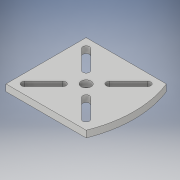
# Autodesk Inventor part: Shoddy Drilling Platform Representation
Saved by Autodesk Inventor 2018 (Build 220112000, 112)
## iProperties
Created: 2018-12-23
Part Number: Shoddy Drilling Platform Representation
Material: Generic
Document SubType Name: Modeling
Designer: Gabriel
Density: 1 g/cm^3
Appearance: Default
Author: Gabriel
Autodesk Inventor part; units mm, degrees
ref_plane "YZ Plane" through (0, 0, 0) normal (1, 0, 0) x (0, 1, 0)
ref_plane "XZ Plane" through (0, 0, 0) normal (0, 1, 0) x (-1, 0, 0)
ref_plane "XY Plane" through (0, 0, 0) normal (0, 0, 1) x (1, 0, 0)
sketch "Sketch1" plane through (0, 0, 0) normal (0, 1, 0) x (-1, 0, 0)
  line L0 (7.0481, 13.5339) -> (-297.7519, 13.5339)
  line L1 (-297.7519, 13.5339) -> (-297.7519, -291.2661)
  line L2 (-297.7519, -291.2661) -> (7.0481, -291.2661)
  line L3 (7.0481, -291.2661) -> (7.0481, 13.5339)
  arc A0 (-297.7519, 13.5339) -> (-297.7519, -291.2661) centre (83.7145, -138.8661) ccw
  point P0 (0, 0)
  dimension "d0" = 304.8
  dimension "d1" = 304.8
  constraints: 8 end point, 2 parallel, 2 point on circle, 1 centre point, 1 horizontal, 1 perpendicular
  measures "d0" distance of L2.end L1.end
  measures "d1" distance of L1.end L0.end
extrude "Extrusion1" add sketch "Sketch1" along normal blind 25.4
sketch "Sketch2" plane through (0, 25.4, 0) normal (0, 1, 0) x (1, 0, 0)
  line L0 (-7.0481, 291.2661) -> (-7.0481, -13.5339) projected
  line L1 (-7.0481, 138.8661) -> (145.3519, 138.8661)
  circle A0 centre (145.3519, 138.8661) radius 19.05
  point P0 (0, 0)
  dimension "d4" = 152.4
  dimension "d5" = 38.1
  constraints: 2 end point, 1 centre point, 1 coincident, 1 horizontal, 1 midpoint
  measures "d4" distance of L1.start L1.end
  measures "d5" diameter of A0
extrude "Extrusion2" cut sketch "Sketch2" against normal blind 50.8
sketch "Sketch3" plane through (0, 25.4, 0) normal (0, 1, 0) x (1, 0, 0)
  line L0 (-7.0481, 291.2661) -> (-7.0481, -13.5339) projected
  line L1 (297.7519, 291.2661) -> (-7.0481, 291.2661) projected
  line L2 (-7.0481, -13.5339) -> (297.7519, 291.2661)
  line L3 (-7.0481, -13.5339) -> (297.7519, -13.5339) projected
  line L4 (-7.0481, 291.2661) -> (297.7519, -13.5339)
  line L5 (-7.0481, -13.5339) -> (28.873, 22.3871)
  line L6 (297.7519, -13.5339) -> (261.8309, 22.3871)
  line L7 (297.7519, 291.2661) -> (261.8309, 255.3451)
  line L8 (-7.0481, 291.2661) -> (28.873, 255.3451)
  line L9 (28.873, 22.3871) -> (261.8309, 22.3871)
  line L10 (261.8309, 22.3871) -> (261.8309, 255.3451)
  line L11 (261.8309, 255.3451) -> (28.873, 255.3451)
  line L12 (28.873, 255.3451) -> (28.873, 22.3871)
  line L13 (28.873, 22.3871) -> (100.715, 94.2292) construction
  line L14 (37.8532, 13.4068) -> (109.6953, 85.2489)
  line L15 (91.7348, 103.2094) -> (19.8927, 31.3674)
  arc A0 (19.8927, 31.3674) -> (37.8532, 13.4068) centre (28.873, 22.3871) ccw
  arc A1 (109.6953, 85.2489) -> (91.7348, 103.2094) centre (100.715, 94.2292) ccw
  line L16 (28.873, 255.3451) -> (100.715, 183.503) construction
  line L17 (19.8927, 246.3648) -> (91.7348, 174.5228)
  line L18 (109.6953, 192.4833) -> (37.8532, 264.3253)
  arc A2 (37.8532, 264.3253) -> (19.8927, 246.3648) centre (28.873, 255.3451) ccw
  arc A3 (91.7348, 174.5228) -> (109.6953, 192.4833) centre (100.715, 183.503) ccw
  line L19 (261.8309, 22.3871) -> (189.9889, 94.2292) construction
  line L20 (270.8112, 31.3674) -> (198.9691, 103.2094)
  line L21 (181.0086, 85.2489) -> (252.8507, 13.4068)
  arc A4 (252.8507, 13.4068) -> (270.8112, 31.3674) centre (261.8309, 22.3871) ccw
  arc A5 (198.9691, 103.2094) -> (181.0086, 85.2489) centre (189.9889, 94.2292) ccw
  line L22 (261.8309, 255.3451) -> (189.9889, 183.503) construction
  line L23 (252.8507, 264.3253) -> (181.0086, 192.4833)
  line L24 (198.9691, 174.5228) -> (270.8112, 246.3648)
  arc A6 (270.8112, 246.3648) -> (252.8507, 264.3253) centre (261.8309, 255.3451) ccw
  arc A7 (181.0086, 192.4833) -> (198.9691, 174.5228) centre (189.9889, 183.503) ccw
  point P0 (0, 0)
  point P1 (64.794, 58.3081)
  point P2 (64.794, 219.424)
  point P3 (225.9099, 58.3081)
  point P4 (225.9099, 219.424)
  dimension "d8" = 50.8
  dimension "d9" = 50.8
  dimension "d10" = 50.8
  dimension "d11" = 50.8
  dimension "d12" = 101.6
  dimension "d13" = 25.4
  dimension "d14" = 101.6
  dimension "d15" = 25.4
  dimension "d16" = 101.6
  dimension "d17" = 25.4
  dimension "d18" = 101.6
  dimension "d19" = 25.4
  constraints: 52 end point, 16 point on circle, 16 tangent, 8 centre point, 8 point on line, 6 parallel, 4 midpoint, 1 horizontal, 1 perpendicular
  measures "d8" distance of L0.end L5.end
  measures "d9" distance of L3.end L6.end
  measures "d10" distance of L1.start L7.end
  measures "d11" distance of L0.start L8.end
  measures "d12" distance of L5.end L13.end
  measures "d13" diameter of A1
  measures "d14" distance of L11.end L16.end
  measures "d15" diameter of A3
  measures "d16" distance of L9.end L19.end
  measures "d17" diameter of A5
  measures "d18" distance of L7.end L22.end
  measures "d19" diameter of A7
extrude "Extrusion3" cut sketch "Sketch3" against normal blind 50.8 contours A2 L18 L11 L4 | L4 L12 L17 A2 | A0 L15 L12 L2 | L2 L9 L14 A0 | A6 L24 L10 L2 | L2 L11 L23 A6 | L11 L18 A3 L4 | L4 A3 L17 L12 | L12 L15 A1 L2 | L2 A1 L14 L9 | A4 L21 L9 L4 | L4 L10 L20 A4 | L10 L24 A7 L2 | L2 A7 L23 L11 | L9 L21 A5 L4 | L4 A5 L20 L10
body "Solid1"
